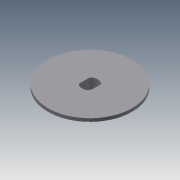
# Autodesk Inventor part: disc_put
Saved by Autodesk Inventor 2014 (Build 180170000, 170)
## iProperties
Created: 2014-09-06
Part Number: disc_put
Material: 一般
Document SubType Name: Modeling
Designer: Hideyuki Takei
Density: 1 g/cm^3
Appearance: 既定
Author: Hideyuki Takei
Autodesk Inventor part; units mm, degrees
ref_plane "YZ Plane" through (0, 0, 0) normal (1, 0, 0) x (0, 1, 0)
ref_plane "XZ Plane" through (0, 0, 0) normal (0, 1, 0) x (-1, 0, 0)
ref_plane "XY Plane" through (0, 0, 0) normal (0, 0, 1) x (1, 0, 0)
sketch "スケッチ1" plane through (0, 0, 0) normal (0, 0, 1) x (1, 0, 0)
  circle A0 centre (0, 0) radius 5
  circle A1 centre (0, 0) radius 3.75
  line L0 (-3.75, 3) -> (-2.75, 3)
  line L1 (-2.75, 3) -> (-2.75, -3)
  line L2 (-2.75, -3) -> (-3.75, -3)
  line L3 (-3.75, -3) -> (-3.75, 3)
  line L4 (3.75, -3) -> (2.75, -3)
  line L5 (2.75, -3) -> (2.75, 3)
  line L6 (2.75, 3) -> (3.75, 3)
  line L7 (3.75, 3) -> (3.75, -3)
  dimension "d0" = 10
  dimension "d1" = 7.5
  dimension "d2" = 5.5
  dimension "d3" = 1
  dimension "d4" = 1
  dimension "d5" = 6
  dimension "d6" = 6
  dimension "d7" = 3
  dimension "d8" = 2.75
  dimension "d17" = 3
  constraints: 16 end point, 4 parallel, 2 centre point, 2 coincident, 2 horizontal, 2 perpendicular
  measures "d0" diameter of A0
  measures "d1" diameter of A1
  measures "d2" distance between parallel lines of L5 L1
  measures "d3" distance of L0.start L0.end
  measures "d4" distance of L5.end L6.end
  measures "d5" distance of L2.end L0.start
  measures "d6" distance of L6.end L4.start
  measures "d7" distance from line of point (0, 0) L0
  measures "d8" horizontal distance of point (0, 0) L0.end
  measures "d17" distance from line of point (0, 0) L6
extrude "押し出し1" add sketch "スケッチ1" against normal blind 5 contours A0 | A1 L5 | L7 L4 L5 A1 | A1 L5 L6 L7 | L1 A1 | A1 L3 L0 L1 | L1 L2 L3 A1
sketch "スケッチ2" plane through (0, 0, 0) normal (0, 0, 1) x (1, 0, 0)
  circle A0 centre (0, 0) radius 20
  circle A1 centre (0, 0) radius 4
  dimension "d11" = 40
  dimension "d14" = 8
  constraints: 2 centre point, 2 coincident
  measures "d11" diameter of A0
  measures "d14" diameter of A1
extrude "押し出し3" add sketch "スケッチ2" against normal blind 1.5
equation "\"d8\" = 0.5 * d2"
